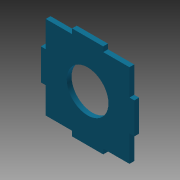
# Autodesk Inventor part: Top
Saved by Autodesk Inventor 2014 SP2 (Build 180246200, 246)
## iProperties
Created: 2014-11-21
Part Number: Top
Material: Generic
Document SubType Name: Modeling
Designer: JLM
Density: 1 g/cm^3
Appearance: Default
Author: JLM
Autodesk Inventor part; units mm, degrees
ref_plane "YZ Plane" through (0, 0, 0) normal (1, 0, 0) x (0, 1, 0)
ref_plane "XZ Plane" through (0, 0, 0) normal (0, 1, 0) x (-1, 0, 0)
ref_plane "XY Plane" through (0, 0, 0) normal (0, 0, 1) x (1, 0, 0)
sketch "Sketch1" plane through (0, 0, 0) normal (0, 0, 1) x (1, 0, 0)
  line L0 (-28.5, -28.5) -> (28.5, -28.5)
  line L1 (28.5, -28.5) -> (28.5, 28.5)
  line L2 (28.5, 28.5) -> (-28.5, 28.5)
  line L3 (-28.5, 28.5) -> (-28.5, -28.5)
  line L4 (-28.5, -28.5) -> (28.5, 28.5) construction
  line L5 (28.5, -28.5) -> (-28.5, 28.5) construction
  point P0 (0, 0)
  dimension "d0" = 57
  dimension "d1" = 57
  constraints: 12 end point, 2 midpoint, 2 parallel, 1 horizontal, 1 perpendicular
  measures "d0" distance of L2.end L1.end
  measures "d1" distance of L1.end L0.end
extrude "Extrusion1" add sketch "Sketch1" against normal blind 2.921
sketch "Sketch2" plane through (0, 0, 0) normal (0, 0, 1) x (1, 0, 0)
  line L0 (-28.5, 28.5) -> (-9.5, 28.5)
  line L1 (-9.5, 28.5) -> (-9.5, 25.5)
  line L2 (-9.5, 25.5) -> (-25.5, 25.5)
  line L3 (-28.5, 22.4359) -> (-28.5, 28.5)
  line L4 (-28.5, 28.5) -> (-22.225, 28.5)
  line L5 (-25.5, 25.5) -> (-25.5, 9.5)
  line L6 (-25.5, 9.5) -> (-28.5, 9.5)
  line L7 (-28.5, 9.5) -> (-28.5, 28.5)
  line L8 (28.5, 28.5) -> (-28.5, 28.5) projected
  line L9 (-28.5, 28.5) -> (-28.5, -28.5) projected
  line L10 (0, 4.0972) -> (0, 8.5289)
  line L11 (-5.3828, 0) -> (-2.3228, 0)
  line L12 (28.5, 28.5) -> (9.5, 28.5)
  line L13 (9.5, 28.5) -> (9.5, 25.5)
  line L14 (9.5, 25.5) -> (25.5, 25.5)
  line L15 (28.5, 22.4359) -> (28.5, 28.5)
  line L16 (28.5, 28.5) -> (22.225, 28.5)
  line L17 (25.5, 25.5) -> (25.5, 9.5)
  line L18 (25.5, 9.5) -> (28.5, 9.5)
  line L19 (28.5, 9.5) -> (28.5, 28.5)
  line L20 (-28.5, -28.5) -> (-9.5, -28.5)
  line L21 (-9.5, -28.5) -> (-9.5, -25.5)
  line L22 (-9.5, -25.5) -> (-25.5, -25.5)
  line L23 (-28.5, -22.4359) -> (-28.5, -28.5)
  line L24 (-28.5, -28.5) -> (-22.225, -28.5)
  line L25 (-25.5, -25.5) -> (-25.5, -9.5)
  line L26 (-25.5, -9.5) -> (-28.5, -9.5)
  line L27 (-28.5, -9.5) -> (-28.5, -28.5)
  line L28 (28.5, -28.5) -> (-28.5, -28.5)
  line L29 (28.5, -28.5) -> (9.5, -28.5)
  line L30 (9.5, -28.5) -> (9.5, -25.5)
  line L31 (9.5, -25.5) -> (25.5, -25.5)
  line L32 (28.5, -22.4359) -> (28.5, -28.5)
  line L33 (28.5, -28.5) -> (22.225, -28.5)
  line L34 (25.5, -25.5) -> (25.5, -9.5)
  line L35 (25.5, -9.5) -> (28.5, -9.5)
  line L36 (28.5, -9.5) -> (28.5, -28.5)
  line L37 (-28.5, -28.5) -> (28.5, -28.5) projected
  line L38 (28.5, -28.5) -> (28.5, 28.5) projected
  point P0 (0, -8.5289)
  dimension "d59" = 3
  dimension "d62" = 3
  dimension "d65" = 19
  dimension "d66" = 19
  dimension "d67" = 19
  dimension "d68" = 19
  dimension "d69" = 19
  dimension "d70" = 19
  dimension "d71" = 19
  dimension "d72" = 19
  dimension "d73" = 19
  dimension "d74" = 19
  dimension "d75" = 19
  dimension "d76" = 19
  constraints: 70 end point, 29 symmetric about line, 5 parallel, 3 perpendicular, 2 collinear, 2 horizontal
  measures "d59" distance of L0.end L1.end
  measures "d62" distance of L5.end L6.end
  measures "d65" distance between parallel lines of L13 L1
  measures "d66" distance between parallel lines of L3 L1
  measures "d67" distance between parallel lines of L38 L13
  measures "d68" distance between parallel lines of L26 L6
  measures "d69" distance between parallel lines of L35 L18
  measures "d70" distance between parallel lines of L8 L6
  measures "d71" distance between parallel lines of L8 L18
  measures "d72" distance between parallel lines of L28 L26
  measures "d73" distance between parallel lines of L37 L35
  measures "d74" distance between parallel lines of L30 L21
  measures "d75" distance between parallel lines of L21 L9
  measures "d76" distance between parallel lines of L38 L30
extrude "Extrusion3" cut sketch "Sketch2" against normal up to next contours L0 L1 L2 L5 L6 L7 L3 | L8 L15 L19 L18 L17 L14 L13 | L26 L25 L22 L21 L20 L9 | L36 L32 L28 L30 L31 L34 L35
hole "Hole1" at (0, 0, 0) direction (0, 0, -1) diameter 25.4 end through all
equation "\"d1\" = d0"
equation "\"d62\" = d59"
equation "\"d68\" = d65"
equation "\"d70\" = d66"
equation "\"d23\" = 0.5 * d0"
equation "\"d53\" = 0.5 * d0"
body "Solid1"
